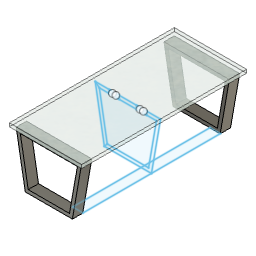
plan (Autodesk Fusion 360 design; units mm, degrees)
Autodesk Fusion 360 part; units mm, degrees
sketch "Sketch1" plane through (0, 0, 0) normal (0, 0, 1) x (1, 0, 0)
  line L0 (-266.7, -609.6) -> (266.7, -609.6)
  line L1 (266.7, -609.6) -> (266.7, 609.6)
  line L2 (266.7, 609.6) -> (-266.7, 609.6)
  line L3 (-266.7, 609.6) -> (-266.7, -609.6)
  dimension "d1" = 533.4
  dimension "d2" = 1219.2
  constraint horizontal L0
  constraint vertical L1
  constraint horizontal L2
  constraint vertical L3
  measures "d1" distance of L0.start L0.end
  measures "d2" distance of L0.start L2.end
extrude "Extrude1" add sketch "Sketch1" along normal blind 25.4 makes body 1
sketch "Sketch2" plane through (0, 0, 0) normal (0, 1, 0) x (1, 0, 0)
  line L0 (-241.9712, 2.2344) -> (240.6288, 2.2344)
  line L1 (240.6288, 2.2344) -> (173.4483, 383.2344)
  line L2 (173.4483, 383.2344) -> (-174.7906, 383.2344)
  line L3 (-174.7906, 383.2344) -> (-241.9712, 2.2344)
  line L4 (-211.7006, 27.6344) -> (210.3583, 27.6344)
  line L5 (210.3583, 27.6344) -> (152.1351, 357.8344)
  line L6 (152.1351, 357.8344) -> (-153.4775, 357.8344)
  line L7 (-153.4775, 357.8344) -> (-211.7006, 27.6344)
  line L8 (-140.3712, 2.2344) -> (-64.6175, 2.2344)
  line L9 (-64.6175, 2.2344) -> (-64.6175, 27.6344)
  line L10 (-64.6175, 27.6344) -> (-140.3712, 27.6344)
  line L11 (-140.3712, 27.6344) -> (-140.3712, 2.2344)
  line L12 (62.8288, 2.2344) -> (139.2321, 2.2344)
  line L13 (139.2321, 2.2344) -> (139.2321, 27.6344)
  line L14 (139.2321, 27.6344) -> (62.8288, 27.6344)
  line L15 (62.8288, 27.6344) -> (62.8288, 2.2344)
  circle A0 centre (-114.9712, 14.9344) radius 3.175
  circle A1 centre (-89.5712, 14.9344) radius 3.175
  circle A2 centre (88.2288, 14.9344) radius 3.175
  circle A3 centre (113.6288, 14.9344) radius 3.175
  line L16 (-241.9712, 2.2344) -> (-211.7006, 27.6344)
  line L17 (-174.7906, 383.2344) -> (-153.4775, 357.8344)
  dimension "d5" = 482.6
  dimension "interiorAngle" = 100
  dimension "d7" = 100
  dimension "d8" = 381
  dimension "d9" = 348.2388
  dimension "d10" = 386.8775
  dimension "tubeWidth" = 25.4
  dimension "d12" = 25.4
  dimension "d14" = 25.4
  dimension "d40" = 80
  dimension "d41" = 305.6126
  dimension "d42" = 422.0589
  dimension "d43" = 335.2939
  dimension "d54" = 25.4
  dimension "d60" = 6.35
  dimension "d85" = 127
  dimension "d86" = 177.8
  dimension "d87" = 25.4
  dimension "d88" = 25.4
  dimension "d89" = 40
  dimension "d90" = 50
  constraint horizontal L0
  constraint parallel L0 L2
  constraint horizontal L4
  constraint parallel L4 L6
  constraint parallel L3 L7
  constraint parallel L1 L5
  constraint horizontal L8
  constraint vertical L9
  constraint horizontal L10
  constraint vertical L11
  constraint coincident L0 L8.start
  constraint horizontal L12
  constraint vertical L13
  constraint horizontal L14
  constraint vertical L15
  constraint coincident L0 L12.start
  constraint coincident L4 L9.end
  measures "d5" distance of L0.start L0.end
  measures "interiorAngle" angle of L2 L3
  measures "d7" angle of L1 L2
  measures "d8" distance of L0 L2
  measures "d9" distance of L1.end L2.end
  measures "d10" distance of L0.end L1.end
  measures "tubeWidth" distance of L3 L7
  measures "d12" distance of L1 L5
  measures "d14" distance of L2 L6
  measures "d40" angle of L4 L7
  measures "d41" distance of L5.end L6.end
  measures "d42" distance of L4.start L4.end
  measures "d43" distance of L4.end L5.end
  measures "d54" distance of L12.start L14.end
  measures "d60" diameter of A3
  measures "d85" horizontal distance of L0.end A3.centre
  measures "d86" distance of A1.centre A2.centre
  measures "d87" distance of A2.centre A3.centre
  measures "d88" distance of A0.centre A1.centre
  measures "d89" angle of L0 L16
  measures "d90" angle of L2 L17
extrude "Extrude2" add sketch "Sketch2" along normal blind 76.2 separate body contours L0 L4 L11 L16 | L3 L7 L16 L17 | L0 L4 L8 L9 L10 L11 | L0 L1 L2 L4 L5 L6 L13 L17 | L0 L4 L9 L15 | L0 L4 L12 L13 L14 L15 | A0 | A1 | A2 | A3 makes body 2
move_body "Move1" bodies 2 to x (1, 0, 0) y (0, 1, 0) z (0, 0, 1) at (0, -584.2, 0)
copy_body "CopyPasteBodies1" bodies 2 makes body 3
move_body "Move2" bodies 3 to x (1, 0, 0) y (0, 1, 0) z (0, 0, 1) at (0, 1092.2, 0)
sketch "Sketch3" plane through (0, 0, 0) normal (0, 0, 1) x (1, 0, 0)
  line L0 (175.1233, 508, -381) -> (98.9233, 508, -381)
  line L1 (98.9233, 508, -381) -> (98.9233, -508, -381)
  line L2 (98.9233, -508, -381) -> (175.1233, -508, -381)
  line L3 (175.1233, -508, -381) -> (175.1233, 508, -381)
  dimension "d26" = 76.2
  dimension "d27" = 1016
extrude "Extrude3" [suppressed]
move_body "Move11" [suppressed]
move_body "Move12" [suppressed]
copy_body "CopyPasteBodies3" [suppressed]
move_body "Move13" [suppressed]
hole "Hole1" [suppressed]
hole "Hole2" [suppressed]
hole "Hole3" [suppressed]
hole "Hole4" [suppressed]
hole "Hole5" [suppressed]
hole "Hole6" [suppressed]
hole "Hole7" [suppressed]
hole "Hole8" [suppressed]
equation "d7 = interiorAngle"
equation "d12 = tubeWidth"
equation "d14 = tubeWidth"
equation "d54 = tubeWidth"
named bodies: "Tabletop", "Legs1", "Legs2", "Strut1", "Strut1 (1)", "Strut2"
